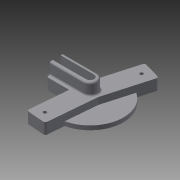
# Autodesk Inventor part: Autonomous - Steering Left
Saved by Autodesk Inventor 2014 (Build 180170000, 170)
## iProperties
Created: 2015-04-23
Part Number: Autonomous - Steering Left
Material: Generic
Document SubType Name: Modeling
Designer: WillHuie
Density: 1 g/cm^3
Appearance: Default
Author: WillHuie
Autodesk Inventor part; units mm, degrees
ref_plane "YZ Plane" through (0, 0, 0) normal (1, 0, 0) x (0, 1, 0)
ref_plane "XZ Plane" through (0, 0, 0) normal (0, 1, 0) x (-1, 0, 0)
ref_plane "XY Plane" through (0, 0, 0) normal (0, 0, 1) x (1, 0, 0)
sketch "Sketch1" plane through (0, 0, 0) normal (0, 1, 0) x (-1, 0, 0)
  line L0 (0, 0) -> (50.8, 0)
  line L1 (0, 0) -> (3.3206, 37.955)
  line L2 (0, 0) -> (38.1, 0) construction
  line L3 (0, 0) -> (-24.2221, -85.5365)
  line L4 (0, 0) -> (88.9, 0) construction
  line L5 (50.8, 0) -> (50.8, 15.24)
  line L6 (50.8, 15.24) -> (16.6315, 15.24)
  line L7 (50.8, 0) -> (50.8, -15.24)
  line L8 (50.8, -15.24) -> (11.5236, -15.24)
  line L9 (-24.2221, -85.5365) -> (-9.5587, -89.6889)
  line L10 (-9.5587, -89.6889) -> (11.5236, -15.24)
  line L11 (-24.2221, -85.5365) -> (-38.8855, -81.3842)
  line L12 (-38.8855, -81.3842) -> (-15.0563, 2.7648)
  line L13 (3.3206, 37.955) -> (-11.8614, 39.2833)
  line L14 (3.3206, 37.955) -> (18.5606, 37.955) construction
  line L15 (-11.8614, 39.2833) -> (-15.0563, 2.7648)
  line L16 (3.3206, 37.955) -> (18.5026, 36.6268)
  line L17 (18.5026, 36.6268) -> (16.6315, 15.24)
  dimension "d0" = 50.8
  dimension "d1" = 38.1
  dimension "d2" = 85
  dimension "d3" = 88.9
  dimension "d4" = 105.811
  dimension "d5" = 15.24
  dimension "d6" = 15.24
  dimension "d7" = 15.24
  dimension "d8" = 15.24
  dimension "d9" = 90
  dimension "d10" = 15.24
  dimension "d11" = 175
  dimension "d12" = 15.24
  constraints: 36 end point, 11 perpendicular, 4 horizontal, 3 equal length
  measures "d0" distance of L0.start L0.end
  measures "d1" distance of L0.start L1.end
  measures "d2" angle of L2 L1
  measures "d3" distance of L0.start L3.end
  measures "d4" angle of L3 L4
  measures "d5" distance of L0.end L5.end
  measures "d6" distance of L0.end L7.end
  measures "d7" distance of L3.end L9.end
  measures "d8" distance of L3.end L11.end
  measures "d9" angle of L11 L12
  measures "d10" distance of L1.end L13.end
  measures "d11" angle of L14 L13
  measures "d12" distance of L1.end L16.end
extrude "Extrusion1" add sketch "Sketch1" along normal blind 16.764
sketch "Sketch2" plane through (0, 16.764, 0) normal (0, 1, 0) x (1, 0, 0)
  circle A0 centre (0, 0) radius 6.096
  dimension "d15" = 12.192
  constraints: 1 centre point, 1 coincident
  measures "d15" diameter of A0
extrude "Extrusion2" cut sketch "Sketch2" against normal blind 16.764
sketch "Sketch3" plane through (0, 16.764, 0) normal (0, 1, 0) x (1, 0, 0)
  circle A0 centre (0, 0) radius 6.096 projected
  line L0 (-50.8, 15.24) -> (-50.8, -15.24) projected
  line L1 (-50.8, -15.24) -> (-16.6315, -15.24) projected
  line L2 (-11.5236, 15.24) -> (-50.8, 15.24) projected
  line L3 (0, 6.096) -> (-50.8, 6.096)
  line L4 (0, -6.096) -> (-50.8, -6.096)
  arc A1 (0, -15.24) -> (0, 15.24) centre (0, 0) ccw
  line L5 (-16.6315, -15.24) -> (0, -15.24)
  line L6 (-11.5236, 15.24) -> (0, 15.24)
  constraints: 8 end point, 4 point on circle, 4 tangent, 2 perpendicular, 2 point on line, 1 centre point, 1 coincident
extrude "Extrusion3" add sketch "Sketch3" along normal blind 17.78 contours A0 L3 L0 L2 L6 A1 L5 L1 L4
fillet "Fillet1" radius 6.096 1 edges at (-25.4, 16.764, -6.096)
fillet "Fillet2" radius 6.096 1 edges at (-25.4, 16.764, 6.096)
fillet "Fillet3" radius 7.62 2 edges at (-4.3105, 18.5495, -4.3105) (-4.3105, 18.5495, 4.3105)
sketch "Sketch4" plane through (11.8614, 0, 39.2833) normal (-0.0871557, 0, 0.9961947) x (0.9961947, 0, 0.0871557)
  line L0 (-30.48, 0) -> (0, 0) projected
  line L1 (0, 0) -> (0, 16.764) projected
  line L2 (-30.48, 16.764) -> (0, 16.764) projected
  line L3 (-30.48, 0) -> (-30.48, 16.764) projected
  point P0 (-15.24, 0)
extrude "Extrusion4" add sketch "Sketch4" along normal blind 17.78
sketch "Sketch5" plane through (9.5587, 0, -89.6889) normal (0.272465, 0, -0.9621657) x (-0.9621657, 0, -0.272465)
  line L0 (-30.48, 0) -> (0, 0) projected
  line L1 (0, 0) -> (0, 16.764) projected
  line L2 (-30.48, 16.764) -> (0, 16.764) projected
  line L3 (-30.48, 0) -> (-30.48, 16.764) projected
  point P0 (-15.24, 0)
extrude "Extrusion5" add sketch "Sketch5" along normal blind 17.78
sketch "Sketch7" plane through (0, 34.544, 0) normal (0, 1, 0) x (1, 0, 0)
  line L0 (-50.8, 15.24) -> (-50.8, 6.096) projected
  line L1 (-50.8, -6.096) -> (-50.8, -15.24) projected
  line L2 (-50.8, -15.24) -> (0, -15.24) projected
  arc A0 (0, -15.24) -> (0, 15.24) centre (0, 0) ccw projected
  line L3 (0, 15.24) -> (-50.8, 15.24) projected
  arc A1 (0, -10.668) -> (0, 10.668) centre (0, 0) ccw
  line L4 (0, 10.668) -> (-50.8, 10.668)
  line L5 (0, -10.668) -> (-50.8, -10.668)
  constraints: 4 end point, 2 midpoint, 2 point on circle, 1 centre point, 1 coincident
extrude "Extrusion6" cut sketch "Sketch7" against normal blind 17.78
fillet "Fillet4" radius 2.54 3 edges at (-25.4, 16.764, 10.668) (10.668, 16.764, 0) (-25.4, 16.764, -10.668)
fillet "Fillet5" radius 2.54 3 edges at (10.668, 34.544, 0) (-25.4, 34.544, -10.668) (-25.4, 34.544, 10.668)
fillet "Fillet6" radius 2.54 1 edges at (-50.8, 8.382, 15.24)
fillet "Fillet7" radius 2.54 1 edges at (-50.8, 8.382, -15.24)
sketch "Sketch9" plane through (0, 0, 0) normal (0, -1, 0) x (1, 0, 0)
  line L0 (15.0563, 2.7648) -> (43.73, -98.4915) projected
  line L1 (15.0563, 2.7648) -> (10.3117, 56.9956) projected
  circle A0 centre (0, 0) radius 6.096 projected
  arc A1 (27.8671, -42.4743) -> (10.9584, 49.604) centre (0, 0) ccw
  point P0 (42.8649, -95.4366)
  point P1 (10.5885, 53.8327)
  dimension "d46" = 101.6
  constraints: 2 point on circle, 2 point on line, 1 centre point, 1 coincident
  measures "d46" diameter of A1
extrude "Extrusion8" add sketch "Sketch9" against normal blind 6.35 contours L1 A1 L0
sketch "Sketch10" plane through (14.4032, 0, -106.7962) normal (0.272465, 0, -0.9621657) x (-0.9621657, 0, -0.272465)
  line L0 (-30.48, 0) -> (0, 0) projected
  line L1 (0, 0) -> (0, 16.764) projected
  line L2 (0, 16.764) -> (-30.48, 16.764) projected
  line L3 (-30.48, 16.764) -> (-30.48, 0) projected
  point P0 (-15.24, 0)
extrude "Extrusion9" cut sketch "Sketch10" against normal blind 30.48
sketch "Sketch11" plane through (10.3117, 0, 56.9956) normal (-0.0871557, 0, 0.9961947) x (0.9961947, 0, 0.0871557)
  line L0 (-30.48, 0) -> (0, 0) projected
  line L1 (0, 0) -> (0, 16.764) projected
  line L2 (0, 16.764) -> (-30.48, 16.764) projected
  line L3 (-30.48, 16.764) -> (-30.48, 0) projected
  point P0 (-15.24, 0)
extrude "Extrusion10" add sketch "Sketch11" along normal blind 20.32
sketch "Sketch12" plane through (0, 16.764, 0) normal (0, 1, 0) x (1, 0, 0)
  circle A0 centre (17.3015, 61.0975) radius 2.54
  circle A1 centre (-5.5344, -63.2584) radius 2.54
  dimension "d55" = 5.08
  dimension "d56" = 5.08
  constraints: 2 centre point
  measures "d55" diameter of A0
  measures "d56" diameter of A1
extrude "Extrusion11" cut sketch "Sketch12" against normal blind 20.32
fillet "Fillet12" radius 3.175 1 edges at (8.5407, 8.382, 77.2383)
fillet "Fillet13" radius 3.175 1 edges at (-21.8233, 8.382, 74.5818)
fillet "Fillet14" radius 3.175 1 edges at (6.0979, 8.382, -77.4675)
fillet "Fillet15" radius 3.175 1 edges at (35.4247, 8.382, -69.1627)
fillet "Fillet16" radius 3.175 1 edges at (15.0563, 11.557, 2.7648)
body "Solid1"
